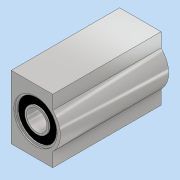
# Autodesk Inventor part: Łożysko liniowe w obudowie SMAG16UU-L
Saved by Autodesk Inventor 2018 (Build 220112000, 112)
## iProperties
Created: 2019-02-01
Part Number: Łożysko liniowe w obudowie SMAG16UU-L
Material: Ogólny
Document SubType Name: Modeling
Designer: Dawid
Density: 1 g/cm^3
Appearance: Aluminium — ciemne
Author: Dawid
Autodesk Inventor part; units mm, degrees
ref_plane "YZ Plane" through (0, 0, 0) normal (1, 0, 0) x (0, 1, 0)
ref_plane "XZ Plane" through (0, 0, 0) normal (0, 1, 0) x (-1, 0, 0)
ref_plane "XY Plane" through (0, 0, 0) normal (0, 0, 1) x (1, 0, 0)
sketch "Szkic1" plane through (0, 0, 0) normal (0, 1, 0) x (-1, 0, 0)
  line L0 (-13.25, 25) -> (19.25, 25)
  line L1 (19.25, 25) -> (19.25, -25)
  line L2 (19.25, -25) -> (-13.25, -25)
  line L3 (-19.25, 25) -> (19.25, -25) construction
  line L4 (19.25, 25) -> (-19.25, -25) construction
  line L5 (19.25, 0) -> (38.5, 0) construction
  line L6 (19.25, 0) -> (0.25, 0)
  line L7 (19.25, 0) -> (38.25, 0) construction
  circle A0 centre (0.25, 0) radius 8
  line L8 (19.25, 25) -> (-13.25, 25)
  line L9 (19.25, 25) -> (51.75, 25) construction
  arc A1 (-19.25, 0) -> (-13.25, -13.9642) centre (0, 0) ccw
  arc A2 (-13.25, 13.9642) -> (-19.25, 0) centre (0, 0) ccw
  line L10 (-13.25, 25) -> (-13.25, 13.9642)
  line L11 (-13.25, -13.9642) -> (-13.25, -25)
  point P0 (0, 0)
  dimension "d1" = 50
  dimension "d4" = 19
  dimension "d5" = 180
  dimension "d6" = 16
  dimension "d7" = 32.5
  dimension "d8" = 180
  constraints: 24 end point, 5 horizontal, 5 midpoint, 4 point on circle, 3 centre point, 3 perpendicular, 2 coincident, 2 collinear, 2 equal length
  measures "d1" distance of L0.end L1.end
  measures "d4" distance of L5.start L6.end
  measures "d5" angle of L6 L7
  measures "d6" diameter of A0
  measures "d7" distance of L0.start L0.end
  measures "d8" angle of L8 L9
extrude "Wyciągnięcie proste1" add sketch "Szkic1" along normal blind 85
sketch "Szkic2" plane through (0, 0, 0) normal (0, -1, 0) x (1, 0, 0)
  circle A0 centre (-0.25, 0) radius 8 projected
  circle A1 centre (-0.25, 0) radius 9.5
  circle A2 centre (-0.25, 0) radius 17
  circle A3 centre (-0.25, 0) radius 15.5
  point P0 (0, 0)
  dimension "d11" = 19
  dimension "d12" = 34
  dimension "d13" = 31
  constraints: 3 centre point, 3 coincident
  measures "d11" diameter of A1
  measures "d12" diameter of A2
  measures "d13" diameter of A3
extrude "Wyciągnięcie proste2" cut sketch "Szkic2" against normal blind 1
sketch "Szkic3" plane through (-0.25, 0, 0) normal (0, -1, 0) x (1, 0, 0)
  circle A0 centre (0, 0) radius 9.5 projected
  circle A1 centre (0, 0) radius 15.5 projected
  point P0 (0.25, 0)
extrude "Wyciągnięcie proste3" cut sketch "Szkic3" against normal blind 2
sketch "Szkic4" plane through (0, 85, 0) normal (0, 1, 0) x (1, 0, 0)
  circle A0 centre (-0.25, 0) radius 8
  circle A1 centre (-0.25, 0) radius 9.5
  circle A2 centre (-0.25, 0) radius 17
  circle A3 centre (-0.25, 0) radius 15.5
  point P0 (0, 0)
  point P1 (0, 0)
  dimension "d18" = 19
  dimension "d19" = 34
  dimension "d20" = 31
  constraints: 4 centre point, 3 coincident
  measures "d18" diameter of A1
  measures "d19" diameter of A2
  measures "d20" diameter of A3
extrude "Wyciągnięcie proste4" cut sketch "Szkic4" against normal blind 1
sketch "Szkic5" plane through (-0.25, 85, 0) normal (0, 1, 0) x (1, 0, 0)
  circle A0 centre (0, 0) radius 9.5 projected
  circle A1 centre (0, 0) radius 15.5 projected
  point P0 (0.25, 0)
extrude "Wyciągnięcie proste5" cut sketch "Szkic5" against normal blind 2
